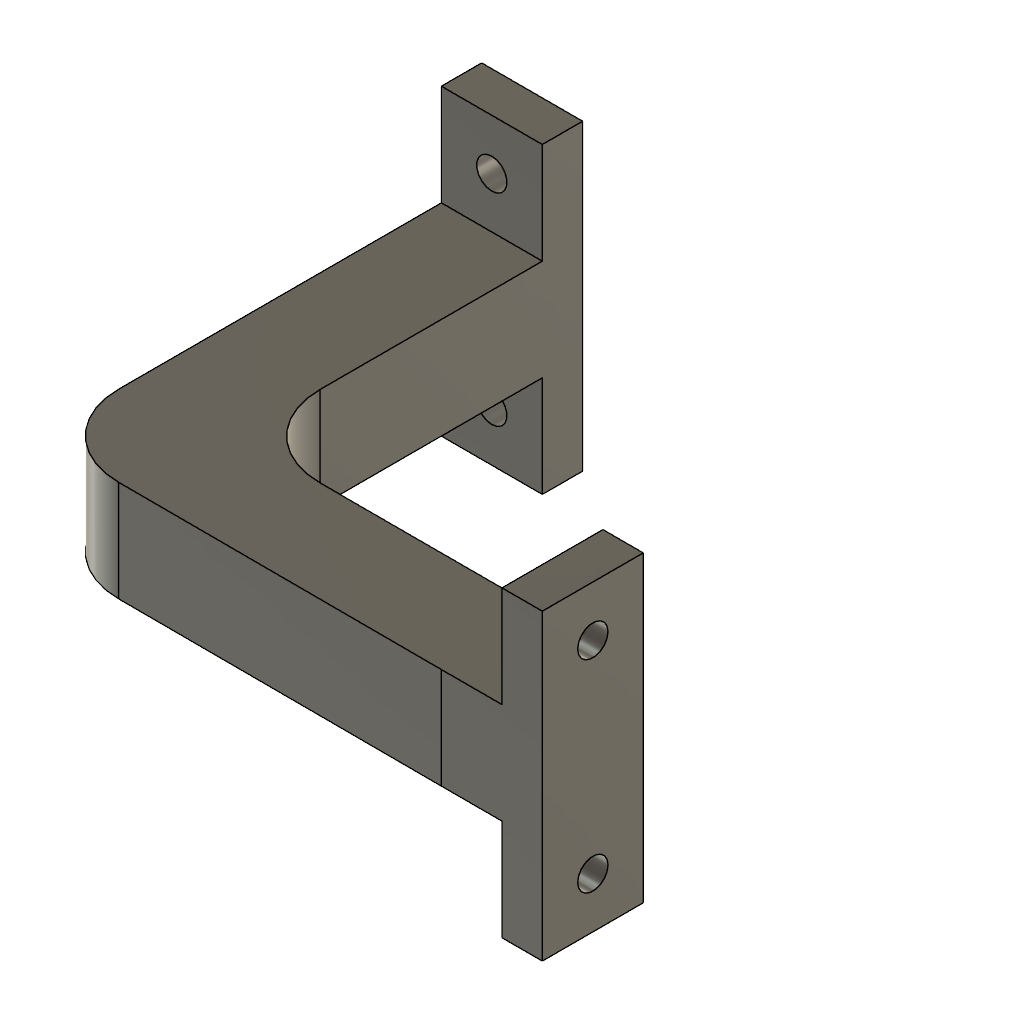
L_Bracket (Autodesk Fusion 360 design; units mm, degrees)
Autodesk Fusion 360 part; units mm, degrees
sketch "Sketch1" plane through (0, 0, 0) normal (0, 0, 1) x (1, 0, 0)
  line L0 (0, 40) -> (10, 40)
  line L1 (10, 40) -> (10, 10)
  line L2 (0, 0) -> (0, 40)
  line L3 (40, 0) -> (40, 10)
  line L4 (40, 10) -> (10, 10)
  line L5 (0, 10) -> (0, 0)
  line L6 (0, 0.1) -> (40, 0)
  dimension "d1" = 10
  dimension "d2" = 40
  dimension "d3" = 40
  dimension "d4" = 10
  constraint horizontal L0
  constraint vertical L1
  constraint vertical L2
  constraint coincident L2.start L5.end
  constraint vertical L3
  constraint horizontal L4
  constraint vertical L5
  constraint coincident L5 L6.start
  measures "d1" distance of L0.start L0.end
  measures "d2" distance of L0.start L2.start
  measures "d3" distance of L2.start L3.start
  measures "d4" distance of L2.start L5.start
extrude "Extrude1" add sketch "Sketch1" along normal blind 10
sketch "Sketch2" plane through (40, 0, 0) normal (1, 0, 0) x (0, 1, 0)
  line L0 (0, 0) -> (10, 0)
  line L1 (10, 0) -> (10, 10)
  line L2 (10, 10) -> (0, 10)
  line L3 (0, 10) -> (0, 0)
  line L4 (0, 20) -> (10, 20)
  line L5 (10, 20) -> (10, -10)
  line L6 (10, -10) -> (0, -10)
  line L7 (0, -10) -> (0, 20)
  dimension "d7" = 10
  dimension "d8" = 30
  constraint horizontal L4
  constraint vertical L5
  constraint horizontal L6
  constraint vertical L7
  measures "d7" distance of L4.start L4.end
  measures "d8" distance of L4.start L6.end
extrude "Extrude2" add sketch "Sketch2" along normal blind 10
sketch "Sketch3" plane through (40, 0, 0) normal (-1, 0, 0) x (0, -1, 0)
  line L0 (-10, 10) -> (0, 10)
  line L1 (0, 10) -> (0, 20)
  line L2 (0, 20) -> (-10, 20)
  line L3 (-10, 20) -> (-10, 10)
extrude "Extrude3" cut sketch "Sketch3" against normal blind 6
move_face "OffsetFaces1" offset -6 1 faces at (40, 3.3333, -6.6667)
sketch "Sketch4" plane through (0, 40, 0) normal (0, 1, 0) x (-1, 0, 0)
  line L0 (-10, 0) -> (0, 0)
  line L1 (0, 0) -> (0, 10)
  line L2 (0, 10) -> (-10, 10)
  line L3 (-10, 10) -> (-10, 0)
  line L4 (-10, 20) -> (0, 20)
  line L5 (0, 20) -> (0, -10)
  line L6 (0, -10) -> (-10, -10)
  line L7 (-10, -10) -> (-10, 20)
  constraint horizontal L4
  constraint vertical L5
  constraint horizontal L6
  constraint vertical L7
extrude "Extrude4" add sketch "Sketch4" along normal blind 4
fillet "Fillet1" radius 8 1 edges at (0, 0.1, 5)
fillet "Fillet2" radius 8 1 edges at (10, 10, 5)
hole "Hole1" at (5.0001, 40, 14.9993) direction (0, 1, 0) diameter 3 end through all
hole "Hole2" at (5.0001, 40, -4.9998) direction (0, 1, 0) diameter 3 end through all
hole "Hole3" at (46, 5.0035, -5.0012) direction (1, 0, 0) diameter 3 end through all
hole "Hole4" at (46, 5.0005, 14.9997) direction (1, 0, 0) diameter 3 end through all
